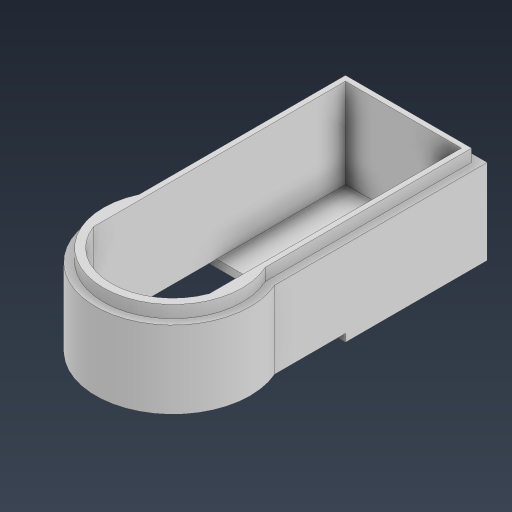
# Autodesk Inventor part: New_base_v3
Saved by Autodesk Inventor 2024 (Build 280153000, 153)
## iProperties
Created: 2025-10-20
Part Number: New_base_v3
Material: Generic
Document SubType Name: Modeling
Designer: Piter
Density: 1 g/cm^3
Appearance: Default
Author: Piter
Autodesk Inventor part; units mm, degrees
ref_plane "YZ Plane" through (0, 0, 0) normal (1, 0, 0) x (0, 1, 0)
ref_plane "XZ Plane" through (0, 0, 0) normal (0, 1, 0) x (-1, 0, 0)
ref_plane "XY Plane" through (0, 0, 0) normal (0, 0, 1) x (1, 0, 0)
sketch "Sketch1" plane through (0, 0, 0) normal (0, 1, 0) x (-1, 0, 0)
  line L0 (-27.5, 47.25) -> (27.5, 47.25)
  line L1 (27.5, 47.25) -> (27.5, -47.25)
  line L2 (27.5, -47.25) -> (-27.5, -47.25)
  line L3 (-27.5, -47.25) -> (-27.5, 47.25)
  line L4 (-27.5, 47.25) -> (27.5, -47.25) construction
  line L5 (27.5, 47.25) -> (-27.5, -47.25) construction
  circle A0 centre (0, 47.25) radius 30
  line L6 (-24.5, 44.25) -> (24.5, 44.25)
  line L7 (24.5, 44.25) -> (24.5, -44.25)
  line L8 (24.5, -44.25) -> (-24.5, -44.25)
  line L9 (-24.5, -44.25) -> (-24.5, 44.25)
  line L10 (-24.5, 44.25) -> (24.5, -44.25) construction
  line L11 (24.5, 44.25) -> (-24.5, -44.25) construction
  line L12 (-22.5, 42.25) -> (22.5, 42.25)
  line L13 (22.5, 42.25) -> (22.5, -42.25)
  line L14 (22.5, -42.25) -> (-22.5, -42.25)
  line L15 (-22.5, -42.25) -> (-22.5, 42.25)
  line L16 (-22.5, 42.25) -> (22.5, -42.25) construction
  line L17 (22.5, 42.25) -> (-22.5, -42.25) construction
  circle A1 centre (0, 47.25) radius 27
  circle A2 centre (0, 47.25) radius 24
  line L18 (22.5, 42.25) -> (22.5, 55.6016)
  line L19 (-22.5, 42.25) -> (-22.5, 55.6016)
  point P0 (0, 0)
  point P1 (27.5, 35.2604)
  point P2 (-27.5, 35.2604)
  point P3 (-22.5, 38.8984)
  point P4 (22.5, 38.8984)
  point P5 (23.8118, 44.25)
  point P6 (22.5, 44.25)
  point P7 (-22.5, 44.25)
  point P8 (-23.8118, 44.25)
  point P9 (24.5, 35.9032)
  point P10 (-24.5, 35.9032)
  dimension "d0" = 55
  dimension "d1" = 94.5
  dimension "d2" = 60
  dimension "d3" = 3
  dimension "d4" = 3
  dimension "d5" = 2
  dimension "d6" = 2
  dimension "d7" = 54
  dimension "d8" = 48
  constraints: 40 end point, 7 midpoint, 7 parallel, 3 centre point, 3 horizontal, 3 perpendicular, 2 coincident, 2 point on circle, 1 vertical
  measures "d0" distance of L1.end L2.end
  measures "d1" distance of L0.end L1.end
  measures "d2" diameter of A0
  measures "d3" distance between parallel lines of L8 L2
  measures "d4" distance between parallel lines of L1 L7
  measures "d5" distance between parallel lines of L13 L7
  measures "d6" distance between parallel lines of L8 L14
  measures "d7" diameter of A1
  measures "d8" diameter of A2
extrude "Extrusion1" add sketch "Sketch1" along normal blind 30 contours A2 L0 A1 | A2 L6 L18 L0 | L0 L18 A2 | L0 A1 L7 L6 A2 | A1 L0 L3 A0 L1 | L0 L1 A0 L7 A1 | A2 L13 L18 L6 | L6 L7 A1 L13 A2 | A1 L9 A0 L3 L0 | L0 A2 L6 L9 A1 | L7 A0 L13 A1 | L19 L6 A2 L0 | L0 A2 L19 | L1 L2 L3 A0 L9 L8 L7 | A1 L15 A0 L9 | L9 L6 A2 L15 A1 | L7 L8 L9 A0 L15 L14 L13 | L19 L15 A2 L6
extrude "Extrusion2" add sketch "Sketch1" along normal blind 34.8 contours A2 L0 A1 | A2 L6 L18 L0 | L0 L18 A2 | L0 A1 L7 L6 A2 | A2 L13 L18 L6 | L6 L7 A1 L13 A2 | L0 A2 L6 L9 A1 | L7 A0 L13 A1 | L19 L6 A2 L0 | L0 A2 L19 | A1 L15 A0 L9 | L9 L6 A2 L15 A1 | L7 L8 L9 A0 L15 L14 L13 | L19 L15 A2 L6
sketch "Sketch2" plane through (0, 0, 0) normal (0, -1, 0) x (1, 0, 0)
  line L0 (-22.5, 55.6016) -> (-22.5, -42.25) projected
  arc A0 (22.5, 55.6016) -> (-22.5, 55.6016) centre (0, 47.25) ccw projected
  line L1 (22.5, -42.25) -> (22.5, 55.6016) projected
  line L2 (-22.5, -42.25) -> (22.5, -42.25) projected
  line L3 (27.5, 35.2604) -> (27.5, -47.25) projected
  arc A1 (27.5, 35.2604) -> (-27.5, 35.2604) centre (0, 47.25) ccw projected
  line L4 (-27.5, -47.25) -> (-27.5, 35.2604) projected
  line L5 (27.5, -47.25) -> (-27.5, -47.25) projected
  line L6 (22.5, -42.25) -> (22.5, 55.6016) projected
  line L7 (27.5, -47.25) -> (-27.5, -47.25)
  line L8 (-27.5, -47.25) -> (-27.5, 7.75)
  line L9 (-27.5, 7.75) -> (27.5, 7.75)
  line L10 (27.5, 7.75) -> (27.5, -47.25)
  point P0 (0, 0)
  dimension "d13" = 55
  dimension "d14" = 55
  constraints: 8 end point, 2 parallel, 1 horizontal, 1 perpendicular
  measures "d13" distance of L8.end L9.end
  measures "d14" distance of L7.end L8.end
extrude "Extrusion3" add sketch "Sketch2" along normal blind 3 contours L9 L1 L2 L0 | L0 L2 L1 L9 L3 L5 L4
body "Solid1"
